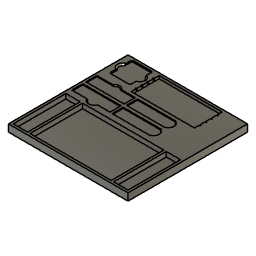
parts-tray v2 (Autodesk Fusion 360 design; units mm, degrees)
Autodesk Fusion 360 part; units mm, degrees
sketch "Sketch1" plane through (0, 0, 0) normal (0, 0, 1) x (1, 0, 0)
  line L0 (-230, 140) -> (20, 140)
  line L1 (20, 140) -> (20, -110)
  line L2 (20, -110) -> (-230, -110)
  line L3 (-230, -110) -> (-230, 140)
  dimension "d1" = 250
  dimension "d2" = 250
  constraint horizontal L0
  constraint vertical L1
  constraint horizontal L2
  constraint vertical L3
  measures "d1" distance of L0.start L0.end
  measures "d2" distance of L0.start L2.end
extrude "Extrude1" add sketch "Sketch1" along normal blind 20 makes body 1
extrude "Extrude2" cut 1 faces at (-146.6667, 56.6667, 20) along direction (0, 0, -1) blind 5 on bodies 1 bodies 1
sketch "Sketch2" plane through (0, 0, 0) normal (0, 0, 1) x (1, 0, 0)
  line L0 (50, 90) -> (90, 90)
  line L1 (90, 90) -> (90, 43)
  line L2 (90, 43) -> (50, 43)
  line L3 (50, 43) -> (50, 90)
  line L4 (105, 90) -> (148, 90)
  line L5 (148, 90) -> (148, 47)
  line L6 (148, 47) -> (105, 47)
  line L7 (105, 47) -> (105, 90)
  dimension "d7" = 40
  dimension "d8" = 47
  dimension "d9" = 43
  dimension "d10" = 43
  constraint horizontal L0
  constraint vertical L1
  constraint horizontal L2
  constraint vertical L3
  constraint horizontal L4
  constraint vertical L5
  constraint horizontal L6
  constraint vertical L7
  measures "d7" distance of L0.start L0.end
  measures "d8" distance of L0.start L2.end
  measures "d9" distance of L4.start L4.end
  measures "d10" distance of L4.start L6.end
extrude "Extrude3" add sketch "Sketch2" along normal blind 5 separate body makes body 2 at (63.3333, 74.3333, 0) makes body 3 at (119.3333, 75.6667, 0)
move_face "MoveFace1" by (-267.0683, 39.8491, 0) 1 faces at (63.3333, 74.3333, 5) on bodies 2
move_body "Move1" bodies 2 to x (1, 0, 0) y (0, 1, 0) z (0, 0, 1) at (-265, 45, 0)
move_body "Move2" bodies 2 to x (1, 0, 0) y (0, 1, 0) z (0, 0, 1) at (0, 0, 10)
extrude "Extrude4" cut 1 faces at (-201.6667, 103.6667, 15) along direction (0, 0, -1) blind 5 on bodies 2 bodies 1 2
move_body "Move3" bodies 3 to x (1, 0, 0) y (0, 1, 0) z (0, 0, 1) at (-321.6, 43, 10)
extrude "Extrude5" cut 1 faces at (-202.2667, 104.3333, 15) along direction (0, 0, -1) blind 5 on bodies 3 bodies 1 3
hole "Hole1" at (-213.0141, 111.8384, 15) direction (0, 0, -1) diameter 16 depth 5 tip angle 180 bodies 1
hole "Hole2" at (-176.4748, 111.6183, 15) direction (0, 0, -1) diameter 16 depth 5 tip angle 180 bodies 1
extrude "Extrude6" add 1 faces at (-187.9333, 109.3079, 10) along direction (0, 0, 1) blind 2 on bodies 1 bodies 1 2 3
box "BoxPrimitive1" cut length 45 width 132 height -6 placed x (0, 1, 0) y (-1, 0, 0) z (0, 0, 1) at (-28, 90, 15) bodies 1
box "BoxPrimitive2" cut length 2 width 2 height -6 placed x (0, -1, 0) y (1, 0, 0) z (0, 0, 1) at (-162, 125.0551, 15) bodies 1
box "BoxPrimitive3" cut length 2 width 2 height -6 placed x (0, 1, 0) y (-1, 0, 0) z (0, 0, 1) at (-160, 111, 15) bodies 1
box "BoxPrimitive4" cut length 2 width 2 height -6 placed x (0, 1, 0) y (-1, 0, 0) z (0, 0, 1) at (-160, 99, 15) bodies 1
extrude "Extrude7" cut 1 faces at (-72, 90, 11) along direction (0, -1, 0) blind 13 on bodies 1 bodies 1
box "BoxPrimitive5" cut length 2 width 2 height -6 placed x (0, 1, 0) y (-1, 0, 0) z (0, 0, 1) at (-160, 87, 15) bodies 1
box "BoxPrimitive6" cut length 2 width 2 height -6 placed x (0, -1, 0) y (1, 0, 0) z (0, 0, 1) at (-28, 125, 15) bodies 1
box "BoxPrimitive7" cut length 2 width 2 height -6 placed x (0, 1, 0) y (-1, 0, 0) z (0, 0, 1) at (-26, 110.9675, 15) bodies 1
box "BoxPrimitive8" cut length 2 width 2 height -6 placed x (0, -1, 0) y (1, 0, 0) z (0, 0, 1) at (-28, 101, 15) bodies 1
box "BoxPrimitive9" cut length 2 width 2 height -6 placed x (0, -1, 0) y (1, 0, 0) z (0, 0, 1) at (-28, 89, 15) bodies 1
box "BoxPrimitive10" cut length 23 width 80 height -2 placed x (0, 1, 0) y (-1, 0, 0) z (0, 0, 1) at (-145, 47, 15) bodies 1
box "BoxPrimitive11" cut length 23 width 80 height -2 placed x (0, 1, 0) y (-1, 0, 0) z (0, 0, 1) at (-145, 17.4919, 15) bodies 1
box "BoxPrimitive12" cut length 23 width 80 height -2 placed x (0, 1, 0) y (-1, 0, 0) z (0, 0, 1) at (-60, 47, 15) bodies 1
box "BoxPrimitive13" cut length 23 width 80 height -2 placed x (0, 1, 0) y (-1, 0, 0) z (0, 0, 1) at (-60, 17, 15) bodies 1
hole "Hole3" at (-182.4877, 65.3169, 15) direction (0, 0, -1) diameter 16 depth 2 tip angle 180 bodies 1
chamfer "Chamfer1" distance 2 angle 45 1 edges at (-182.4877, 73.3169, 15) on bodies 1
hole "Hole4" at (-182.4399, 22.4151, 15) direction (0, 0, -1) diameter 21 depth 2 tip angle 180 bodies 1
chamfer "Chamfer2" distance 2 angle 45 1 edges at (-182.4399, 11.9151, 15) on bodies 1
hole "Hole5" at (-63.7534, 58.6472, 15) direction (0, 0, -1) diameter 21 depth 2 tip angle 180 bodies 1
hole "Hole6" at (-64.7459, 28.6034, 15) direction (0, 0, -1) diameter 21 depth 2 tip angle 180 bodies 1
chamfer "Chamfer3" distance 1 angle 45 1 edges at (-53.2534, 58.6472, 15) on bodies 1
chamfer "Chamfer4" distance 1 angle 45 1 edges at (-54.2459, 28.6034, 15) on bodies 1
chamfer "Chamfer5" distance 3 angle 45 1 edges at (-168.4748, 111.6183, 15) on bodies 1
chamfer "Chamfer6" distance 3 angle 45 1 edges at (-221.0141, 111.8384, 15) on bodies 1
box "BoxPrimitive14" cut length 110 width 240 height -10 placed x (0, 1, 0) y (-1, 0, 0) z (0, 0, 1) at (15, -105, 15) bodies 1
box "BoxPrimitive15" add length 110 width 5 height 10 placed x (0, -1, 0) y (1, 0, 0) z (0, 0, 1) at (-195, 5, 5) bodies 1
box "BoxPrimitive16" add length 110 width 5 height 10 placed x (0, -1, 0) y (1, 0, 0) z (0, 0, 1) at (-20, 5, 5) bodies 1
